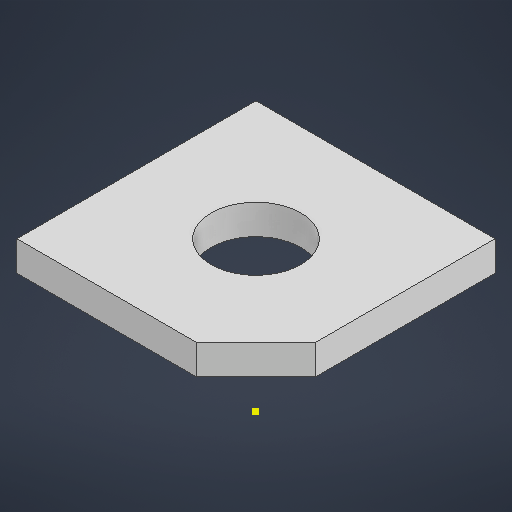
# Autodesk Inventor part: Test
Saved by Autodesk Inventor 2026.1 (Build 301233020, 233B)
## iProperties
Created: 2025-10-22
Part Number: Test
Material: Ogólny
Document SubType Name: Modeling
Designer: obiwa
Density: 1 g/cm^3
Appearance: Domyślna
Author: obiwa
Autodesk Inventor part; units mm, degrees
ref_plane "YZ Plane" through (0, 0, 0) normal (1, 0, 0) x (0, 1, 0)
ref_plane "XZ Plane" through (0, 0, 0) normal (0, 1, 0) x (-1, 0, 0)
ref_plane "XY Plane" through (0, 0, 0) normal (0, 0, 1) x (1, 0, 0)
sketch "Szkic1" plane through (0, 0, 0) normal (0, 1, 0) x (-1, 0, 0)
  point P0 (0, 0)
sketch "Szkic2" plane through (0, 0, 0) normal (0, 1, 0) x (-1, 0, 0)
  line L0 (0, 0) -> (80, 0)
  line L1 (80, 0) -> (80, -80)
  line L2 (80, -80) -> (0, -80)
  line L3 (0, -80) -> (0, 0)
  circle A0 centre (40, -40) radius 15
  line L4 (20, 0) -> (0, -20)
  dimension "d0" = 80
  dimension "d1" = 80
  dimension "d2" = 30
  dimension "d3" = 40
  dimension "d4" = 40
  dimension "d5" = 20
  dimension "d6" = 20
  constraints: 10 end point, 2 parallel, 2 point on line, 1 centre point, 1 horizontal, 1 perpendicular
  measures "d0" distance of L0.end L1.end
  measures "d1" distance of L0.start L0.end
  measures "d2" diameter of A0
  measures "d3" distance from line of L1 A0.centre
  measures "d4" distance from line of A0.centre L0
  measures "d5" distance of L0.start L4.start
  measures "d6" distance of L4.end L0.start
extrude "Wyciągnięcie proste1" add sketch "Szkic2" along normal blind 10 contours L0 L1 L2 L3 L4
